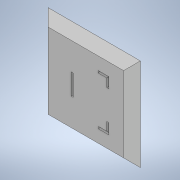
# Autodesk Inventor part: clear-square-outlined
Saved by Autodesk Inventor 2021 (Build 250183000, 183)
## iProperties
Created: 2020-12-08
Part Number: clear-square-outlined
Material: Generic
Document SubType Name: Modeling
Designer: Luke Kamols
Density: 1 g/cm^3
Appearance: Default
Author: Luke Kamols
Autodesk Inventor part; units mm, degrees
ref_plane "YZ Plane" through (0, 0, 0) normal (1, 0, 0) x (0, 1, 0)
ref_plane "XZ Plane" through (0, 0, 0) normal (0, 1, 0) x (-1, 0, 0)
ref_plane "XY Plane" through (0, 0, 0) normal (0, 0, 1) x (1, 0, 0)
sketch "Sketch1" plane through (0, 0, 0) normal (0, 0, 1) x (1, 0, 0)
  line L0 (0, 0) -> (44, 0)
  line L1 (44, 0) -> (44, 44)
  line L2 (44, 44) -> (0, 44)
  line L3 (0, 44) -> (0, 0)
  dimension "d0" = 44
  dimension "d1" = 44
  constraints: 8 end point, 2 parallel, 1 horizontal, 1 perpendicular
  measures "d0" distance of L2.end L1.end
  measures "d1" distance of L1.end L0.end
extrude "Extrusion1" add sketch "Sketch1" along normal blind 4
chamfer "Chamfer1" distance 4 angle 45 4 edges at (22, 44, 4) (44, 22, 4) (22, 0, 4) (0, 22, 4)
sketch "Sketch2" plane through (0, 0, 4) normal (0, 0, 1) x (1, 0, 0)
  line L0 (40, 4) -> (4, 4) projected
  line L1 (22, 4) -> (22, 40)
  line L2 (4, 40) -> (40, 40) projected
  line L3 (22, 40) -> (22, 39)
  line L4 (22, 39) -> (15, 39)
  line L5 (15, 39) -> (15, 5)
  line L6 (15, 5) -> (23, 5)
  line L7 (22, 39) -> (23, 39)
  line L8 (23, 39) -> (23, 34)
  line L9 (23, 34) -> (33, 34)
  line L10 (23, 5) -> (23, 10)
  line L11 (23, 10) -> (33, 10)
  line L12 (33, 10) -> (33, 34)
  line L13 (33, 34) -> (32, 34)
  line L14 (32, 33) -> (32, 29)
  line L15 (32, 29) -> (33, 29)
  line L16 (32, 33) -> (28, 33)
  line L17 (28, 33) -> (28, 34)
  line L18 (33, 10) -> (28, 10)
  line L19 (28, 10) -> (28, 11)
  line L20 (28, 11) -> (32, 11)
  line L21 (32, 11) -> (32, 15)
  line L22 (32, 15) -> (33, 15)
  line L23 (15, 22) -> (16, 22)
  line L24 (16, 22) -> (16, 27)
  line L25 (16, 27) -> (15, 27)
  line L26 (16, 22) -> (16, 17)
  line L27 (16, 17) -> (15, 17)
  point P0 (0, 0)
  dimension "d7" = 1
  dimension "d8" = 7
  dimension "d9" = 34
  dimension "d10" = 8
  dimension "d11" = 1
  dimension "d12" = 5
  dimension "d13" = 10
  dimension "d14" = 5
  dimension "d15" = 10
  dimension "d19" = 5
  dimension "d20" = 1
  dimension "d21" = 4
  dimension "d22" = 4
  dimension "d23" = 1
  dimension "d24" = 5
  dimension "d25" = 5
  constraints: 52 end point, 13 perpendicular, 6 point on line, 5 midpoint, 3 horizontal, 2 vertical, 1 parallel
  measures "d7" distance of L1.end L3.end
  measures "d8" distance of L3.end L4.end
  measures "d9" distance of L4.end L5.end
  measures "d10" distance of L5.end L6.end
  measures "d11" distance of L3.end L7.end
  measures "d12" distance of L7.end L8.end
  measures "d13" distance of L8.end L9.end
  measures "d14" distance of L6.end L10.end
  measures "d15" distance of L10.end L11.end
  measures "d19" distance of L11.end L18.end
  measures "d20" distance of L18.end L19.end
  measures "d21" distance of L19.end L20.end
  measures "d22" distance of L20.end L21.end
  measures "d23" distance of L23.start L23.end
  measures "d24" distance of L23.end L24.end
  measures "d25" distance of L23.end L26.end
extrude "Extrusion2" cut sketch "Sketch2" against normal blind 0.5 contours L5 L23 L26 L27 | L25 L24 L23 L5 | L19 L20 L21 L22 L12 L11 | L9 L12 L15 L14 L16 L17
chamfer "Chamfer2" distance 0.5 angle 45 6 edges at (28, 33.5, 3.5) (30, 33, 3.5) (32, 31, 3.5) (32.5, 29, 3.5) (33, 31.5, 3.5) (30.5, 34, 3.5)
chamfer "Chamfer3" distance 0.5 angle 45 10 edges at (28, 10.5, 3.5) (30.5, 10, 3.5) (32, 13, 3.5) (30, 11, 3.5) (32.5, 15, 3.5) (33, 12.5, 3.5) (15.5, 17, 3.5) (16, 22, 3.5) (15.5, 27, 3.5) (15, 22, 3.5)
body "Solid1"
